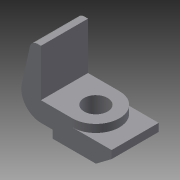
# Autodesk Inventor part: 5.4
Saved by Autodesk Inventor 2015 SP2 (Build 190223200, 223)
## iProperties
Created: 2015-09-23
Part Number: 5.4
Material: Generic
Document SubType Name: Modeling
Designer: KC-019
Density: 1 g/cm^3
Appearance: Default
Author: KC-019
Autodesk Inventor part; units mm, degrees
ref_plane "YZ Plane" through (0, 0, 0) normal (1, 0, 0) x (0, 1, 0)
ref_plane "XZ Plane" through (0, 0, 0) normal (0, 1, 0) x (-1, 0, 0)
ref_plane "XY Plane" through (0, 0, 0) normal (0, 0, 1) x (1, 0, 0)
sketch "Sketch1" plane through (0, 0, 0) normal (0, 0, 1) x (1, 0, 0)
  line L0 (0, 0) -> (0, 76.2)
  line L1 (0, 0) -> (50.8, 0)
  line L2 (50.8, 0) -> (50.8, -12.7)
  line L3 (50.8, -12.7) -> (114.3, -12.7)
  line L4 (114.3, -12.7) -> (114.3, -25.4)
  line L5 (0, 76.2) -> (-5.5192, 76.2)
  arc A0 (-5.5192, 76.2) -> (-17.9219, 66.232) centre (-5.5192, 63.5) ccw
  arc A1 (-31.0067, 6.83) -> (0, -31.75) centre (0, 0) ccw
  line L6 (-17.9219, 66.232) -> (-31.0067, 6.83)
  line L7 (0, -31.75) -> (19.05, -31.75)
  line L8 (6.35, -31.1085) -> (6.35, -31.75)
  line L9 (19.05, -31.75) -> (19.05, -44.45)
  line L10 (19.05, -44.45) -> (88.9, -44.45)
  line L11 (88.9, -44.45) -> (114.3, -25.4)
  dimension "d0" = 76.2
  dimension "d1" = 50.8
  dimension "d2" = 12.7
  dimension "d3" = 63.5
  dimension "d4" = 12.7
  dimension "d13" = 19.05
  dimension "d15" = 12.7
  dimension "d16" = 69.85
  dimension "d17" = 31.75
  dimension "d18" = 59.402
  constraints: 24 end point, 5 point on circle, 4 horizontal, 4 tangent, 3 perpendicular, 3 vertical, 2 centre point, 1 coincident
  measures "d0" distance of L0.start L0.end
  measures "d1" distance of L0.start L1.end
  measures "d2" distance of L1.end L2.end
  measures "d3" distance of L2.end L3.end
  measures "d4" distance of L3.end L4.end
  measures "d13" distance of L7.start L7.end
  measures "d15" distance of L7.end L9.end
  measures "d16" distance of L9.end L10.end
  measures "d17" radius of A1
  measures "d18" vertical distance of L6.start L6.end
extrude "Extrusion1" add sketch "Sketch1" against normal blind 76.2
sketch "Sketch2" plane through (0, 0, 0) normal (0, 1, 0) x (1, 0, 0)
  line L0 (50.8, 0) -> (50.8, 76.2) projected
  circle A0 centre (50.8, 38.1) radius 38.1
  point P0 (0, 0)
  constraints: 1 midpoint, 1 vertical alignment, 2 other
extrude "Extrusion2" add sketch "Sketch2" against normal blind 12.7
sketch "Sketch3" plane through (0, 0, 0) normal (0, 1, 0) x (1, 0, 0)
  arc A0 (50.8, 0) -> (50.8, 76.2) centre (50.8, 38.1) ccw projected
  circle A1 centre (50.8, 38.1) radius 19.05
  point P0 (0, 0)
  dimension "d24" = 38.1
  constraints: 1 centre point, 1 coincident
  measures "d24" diameter of A1
extrude "Extrusion3" cut sketch "Sketch3" against normal through all
body "Solid1"
